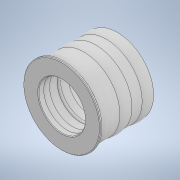
# Autodesk Inventor part: DustPortConvertorShort
Saved by Autodesk Inventor 2022 (Build 260153000, 153)
## iProperties
Created: 2021-11-07
Part Number: DustPortConvertorShort
Material: Generic
Document SubType Name: Modeling
Designer: dangl
Density: 1 g/cm^3
Appearance: Default
Author: dangl
Autodesk Inventor part; units mm, degrees
ref_plane "YZ Plane" through (0, 0, 0) normal (1, 0, 0) x (0, 1, 0)
ref_plane "XZ Plane" through (0, 0, 0) normal (0, 1, 0) x (-1, 0, 0)
ref_plane "XY Plane" through (0, 0, 0) normal (0, 0, 1) x (1, 0, 0)
sketch "Sketch1" plane through (0, 0, 0) normal (0, 1, 0) x (-1, 0, 0)
  line L0 (0, 0) -> (0, -30)
  line L1 (0, 0) -> (-28.5, 0)
  line L2 (-28.5, -45) -> (-25.5, -45)
  line L3 (-25.5, -45) -> (-18, -25)
  line L4 (-18, -25) -> (-18.1552, -17.2395)
  arc A0 (-28.5, -35.3953) -> (-28.5, -45) centre (-13.5, -40.1977) ccw
  arc A1 (-28.5, -17.6977) -> (-28.5, -27.3023) centre (-13.5, -22.5) ccw
  line L5 (-28.5, -27.3023) -> (-28.5, -35.3953)
  line L6 (-28.5, -9.6047) -> (-28.5, -17.6977)
  arc A2 (-18.1552, -17.2395) -> (-18.2054, -14.7277) centre (-19, -16) ccw
  line L7 (-18.2054, -14.7277) -> (-18.326, -8.6999)
  line L8 (-30.5, 0) -> (-30.5, -2)
  line L9 (-30.5, -2) -> (-28.75, -2)
  line L10 (-28.5, 0) -> (-30.5, 0)
  line L11 (-28.5, -2.25) -> (-28.5, -9.6047)
  arc A3 (-28.5, -2.25) -> (-28.75, -2) centre (-28.75, -2.25) ccw
  arc A4 (-18.326, -8.6999) -> (-18.4158, -4.2121) centre (-25, -6.5886) ccw
  line L12 (-18.4158, -4.2121) -> (-18.5, 0)
  dimension "d0" = 30
  dimension "d13" = 3
  dimension "d14" = 25
  dimension "d15" = 45
  dimension "d16" = 18
  dimension "d17" = 18.5
  dimension "d22" = 22.5
  dimension "d25" = 16
  dimension "d26" = 19
  dimension "d27" = 3
  dimension "d28" = 28.5
  dimension "d32" = 2
  dimension "d33" = 2
  dimension "d34" = 0.25
  dimension "d37" = 25
  constraints: 26 end point, 10 point on circle, 5 centre point, 5 perpendicular, 2 horizontal, 2 tangent, 2 vertical, 1 collinear, 1 point on line
  measures "d0" distance of L0.start L0.end
  measures "d13" distance of L2.start L2.end
  measures "d14" vertical distance of L0.start L3.end
  measures "d15" distance between parallel lines of L1 L2
  measures "d16" distance from line of L0 L3.end
  measures "d17" distance of L0.start L12.end
  measures "d22" distance from line of L1 A1.centre
  measures "d25" vertical distance of L0.start A2.centre
  measures "d26" distance from line of L0 A2.centre
  measures "d27" diameter of A2
  measures "d28" distance between parallel lines of L0 L6
  measures "d32" distance between parallel lines of L10 L9
  measures "d33" distance from line of L1.end L8
  measures "d34" radius of A3
  measures "d37" distance from line of L0 A4.centre
revolve "Revolution1" add sketch "Sketch1" angle 360 about axis through (0, 0, 0) along (0, 0, -1)
fillet "Fillet1" radius 0.5 1 edges at (-18.5, 0, 0)
fillet "Fillet2" radius 2 1 edges at (-25.5, 0, -45)
fillet "Fillet3" radius 1 1 edges at (-28.5, 0, -45)
fillet "Fillet4" radius 0.5 2 edges at (-30.5, 0, -2) (-30.5, 0, 0)
fillet "Fillet5" radius 10 1 edges at (-18, 0, -25)
equation "\"d22\" = 0.5 * d15"
body "Solid1"
